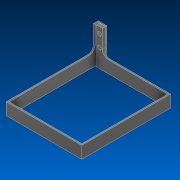
# Autodesk Inventor part: Top Battery Holder
Saved by Autodesk Inventor 2022.2 (Build 262287000, 287)
## iProperties
Created: 2022-04-18
Part Number: Top Battery Holder
Material: PET Plastic
Document SubType Name: Modeling
Designer: omard
Density: 1.541 g/cm^3
Appearance: Smooth - Black
Author: omard
Autodesk Inventor part; units mm, degrees
ref_plane "YZ Plane" through (0, 0, 0) normal (1, 0, 0) x (0, 1, 0)
ref_plane "XZ Plane" through (0, 0, 0) normal (0, 1, 0) x (-1, 0, 0)
ref_plane "XY Plane" through (0, 0, 0) normal (0, 0, 1) x (1, 0, 0)
sketch "Sketch1" plane through (0, 0, 0) normal (0, 1, 0) x (-1, 0, 0)
  line L0 (-76.2, 90.17) -> (76.2, 90.17)
  line L1 (76.2, 90.17) -> (76.2, -90.17)
  line L2 (76.2, -90.17) -> (-76.2, -90.17)
  line L3 (-76.2, -90.17) -> (-76.2, 90.17)
  line L4 (-76.2, 90.17) -> (76.2, -90.17) construction
  line L5 (76.2, 90.17) -> (-76.2, -90.17) construction
  line L6 (-79.375, -93.345) -> (79.375, -93.345)
  line L7 (79.375, -93.345) -> (79.375, 93.345)
  line L8 (79.375, 93.345) -> (-79.375, 93.345)
  line L9 (-79.375, 93.345) -> (-79.375, -93.345)
  line L10 (-79.375, -93.345) -> (79.375, 93.345) construction
  line L11 (79.375, -93.345) -> (-79.375, 93.345) construction
  line L12 (79.375, -93.345) -> (79.375, -99.949)
  line L13 (79.375, -99.949) -> (60.96, -99.949)
  line L14 (60.96, -99.949) -> (60.96, -96.774)
  line L15 (76.2, -93.345) -> (76.2, -96.774)
  line L16 (76.2, -96.774) -> (60.96, -96.774)
  line L17 (76.2, -90.17) -> (76.2, -93.345)
  line L18 (73.66, -90.17) -> (73.66, -93.345)
  line L19 (73.66, -93.345) -> (60.96, -93.345)
  line L20 (60.96, -93.345) -> (60.96, -96.52)
  line L21 (60.96, -96.52) -> (73.66, -96.52)
  line L22 (73.66, -96.52) -> (73.66, -93.345)
  point P0 (0, 0)
  dimension "d2" = 152.4
  dimension "d3" = 180.34
  dimension "d29" = 3.175
  dimension "d30" = 3.175
  dimension "d31" = 2.54
  dimension "d32" = 0.254
  dimension "d33" = 12.7
  constraints: 46 end point, 7 perpendicular, 6 parallel, 4 midpoint, 3 horizontal, 3 point on line, 3 vertical, 2 equal length, 1 collinear
  measures "d2" distance of L1.end L2.end
  measures "d3" distance of L2.end L0.start
  measures "d29" distance between parallel lines of L2 L6
  measures "d30" distance between parallel lines of L1 L7
  measures "d31" distance between parallel lines of L17 L18
  measures "d32" distance between parallel lines of L21 L16
  measures "d33" distance of L20.end L21.end
extrude "Extrusion1" add sketch "Sketch1" along normal blind 25.4 contours L3 L2 L18 L6 L9 L8 L7 L17 L1 L0 | L6 L12 L13 L14 L16 L15 | L22 L21 L20 L6
sketch "Sketch5" plane through (0, 25.4, 0) normal (0, 1, 0) x (1, 0, 0)
  line L0 (-76.2, -90.17) -> (-76.2, 96.774) projected
  line L1 (-76.2, 96.774) -> (-60.96, 96.774) projected
  line L2 (-60.96, 96.774) -> (-60.96, 99.949) projected
  line L3 (-60.96, 99.949) -> (-79.375, 99.949) projected
  line L4 (-79.375, 99.949) -> (-79.375, -93.345) projected
  line L5 (-79.375, -93.345) -> (79.375, -93.345) projected
  line L6 (79.375, -93.345) -> (79.375, 93.345) projected
  line L7 (79.375, 93.345) -> (-60.96, 93.345) projected
  line L8 (-60.96, 93.345) -> (-60.96, 96.52) projected
  line L9 (-60.96, 96.52) -> (-73.66, 96.52) projected
  line L10 (-73.66, 96.52) -> (-73.66, 90.17) projected
  line L11 (-73.66, 90.17) -> (76.2, 90.17) projected
  line L12 (76.2, 90.17) -> (76.2, -90.17) projected
  line L13 (76.2, -90.17) -> (-76.2, -90.17) projected
  line L14 (-60.96, 99.949) -> (-79.375, 99.949) projected
  line L15 (-79.375, 99.949) -> (-79.375, -93.345) projected
  line L16 (-60.96, 99.949) -> (-79.375, 99.949)
  line L17 (-79.375, 99.949) -> (-79.375, 96.774)
  line L18 (-79.375, 96.774) -> (-60.96, 96.774)
  line L19 (-60.96, 96.774) -> (-60.96, 99.949)
  line L20 (-60.96, 93.345) -> (-60.96, 96.52) projected
  line L21 (-73.66, 96.52) -> (-73.66, 90.17) projected
  line L22 (-60.96, 96.52) -> (-73.66, 96.52)
  line L23 (-73.66, 96.52) -> (-73.66, 90.17)
  line L24 (-73.66, 90.17) -> (-60.96, 90.17)
  line L25 (-60.96, 90.17) -> (-60.96, 96.52)
  line L26 (-76.2, -90.17) -> (-76.2, 96.774) projected
  line L27 (-79.375, 96.774) -> (-76.2, 96.774)
  line L28 (-76.2, 96.774) -> (-76.2, 90.17)
  line L29 (-76.2, 90.17) -> (-79.375, 90.17)
  line L30 (-79.375, 90.17) -> (-79.375, 96.774)
  point P0 (0, 0)
  point P1 (-60.96, 93.345)
  constraints: 24 end point, 6 parallel, 3 horizontal, 3 perpendicular, 3 point on line, 1 collinear
extrude "Extrusion4" add sketch "Sketch5" along normal blind 50.8 contours L29 L4 L18 L0 | L18 L4 L3 L2 L1 | L11 L10 L9 L8 L25
sketch "Sketch6" plane through (-73.66, 0, -90.17) normal (0, 0, 1) x (1, 0, 0)
  line L0 (0, 76.2) -> (12.7, 76.2) projected
  line L1 (12.7, 25.4) -> (12.7, 76.2) projected
  point P0 (73.66, 0)
  point P1 (6.35, 63.5)
  point P2 (6.35, 38.1)
  dimension "d36" = 12.7
  dimension "d37" = 25.4
  dimension "d38" = 6.35
  constraints: 1 vertical alignment
  measures "d36" distance from line of L0 point (6.35, 63.5)
  measures "d37" distance of point (6.35, 38.1) point (6.35, 63.5)
  measures "d38" distance from line of L1 point (6.35, 63.5)
hole "Hole2" at (-67.31, 63.5, -90.17) at (-67.31, 38.1, -90.17) direction (0, 0, -1) diameter 4.445 end through all start extended yes counterbore diameter 8.89 counterbore depth 2.54
fillet "Fillet3" radius 12.7 2 edges at (-60.96, 25.4, -91.7575) (-77.7875, 25.4, -90.17)
fillet "Fillet3" radius 12.7 1 edges at (-60.96, 12.7, -93.345)
body "Solid1"
